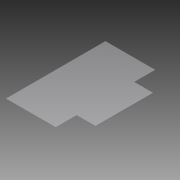
# Autodesk Inventor part: Plexiglass Mounting Sheet
Saved by Autodesk Inventor 2015 (Build 190159000, 159)
## iProperties
Created: 2015-01-31
Part Number: Plexiglass Mounting Sheet
Material: Acrylic, Clear
Document SubType Name: Modeling
Designer: Bhaskar
Density: 1.19 g/cm^3
Appearance: Transparent - Clear
Author: Bhaskar
Autodesk Inventor part; units mm, degrees
ref_plane "YZ Plane" through (0, 0, 0) normal (1, 0, 0) x (0, 1, 0)
ref_plane "XZ Plane" through (0, 0, 0) normal (0, 1, 0) x (-1, 0, 0)
ref_plane "XY Plane" through (0, 0, 0) normal (0, 0, 1) x (1, 0, 0)
sketch "Sketch1" plane through (0, 0, 0) normal (0, 1, 0) x (-1, 0, 0)
  line L0 (0, 0) -> (245, 0)
  line L1 (245, 0) -> (245, -355.6)
  line L2 (245, -355.6) -> (0, -355.6)
  line L3 (0, -355.6) -> (0, 0)
  line L4 (0, -355.6) -> (67.5, -355.6)
  line L5 (67.5, -355.6) -> (67.5, -280.6)
  line L6 (67.5, -280.6) -> (0, -280.6)
  line L7 (0, -280.6) -> (0, -355.6)
  line L8 (0, 0) -> (67.4878, 0)
  line L9 (67.4878, 0) -> (67.4878, -75.0062)
  line L10 (67.4878, -75.0062) -> (0, -75.0062)
  line L11 (0, -75.0062) -> (0, 0)
  dimension "d0" = 245
  dimension "d1" = 355.6
  dimension "d2" = 67.5
  dimension "d3" = 75
  dimension "d4" = 67.4878
  dimension "d5" = 75.0062
  constraints: 24 end point, 6 parallel, 3 horizontal, 3 perpendicular
  measures "d0" distance of L1.end L2.end
  measures "d1" distance of L0.end L1.end
  measures "d2" distance of L6.end L5.end
  measures "d3" distance of L5.end L4.end
  measures "d4" distance of L9.end L10.end
  measures "d5" distance of L8.end L9.end
extrude "Extrusion1" add sketch "Sketch1" along normal blind 2.5 contours L0 L1 L2 L5 L6 L3 L10 L9
body "Solid1"
